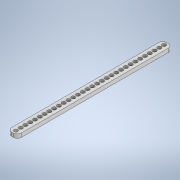
# Autodesk Inventor part: rearLeg_bot
Saved by Autodesk Inventor 2020 (Build 240168000, 168)
## iProperties
Created: 2019-04-04
Part Number: rearLeg_bot
Material: Generic
Document SubType Name: Modeling
Designer: mfans
Density: 1 g/cm^3
Appearance: Default
Author: mfans
Autodesk Inventor part; units mm, degrees
ref_plane "YZ Plane" through (0, 0, 0) normal (1, 0, 0) x (0, 1, 0)
ref_plane "XZ Plane" through (0, 0, 0) normal (0, 1, 0) x (-1, 0, 0)
ref_plane "XY Plane" through (0, 0, 0) normal (0, 0, 1) x (1, 0, 0)
sketch "Sketch1" plane through (0, 0, 0) normal (0, 1, 0) x (-1, 0, 0)
  line L0 (5, 80) -> (-5, 80)
  line L1 (-5, 80) -> (-5, -80)
  line L2 (-5, -80) -> (5, -80)
  line L3 (5, -80) -> (5, 80)
  line L4 (5, 80) -> (-5, -80) construction
  line L5 (-5, 80) -> (5, -80) construction
  point P0 (0, 0)
  dimension "d0" = 10
  dimension "d1" = 160
  constraints: 12 end point, 2 midpoint, 2 parallel, 1 horizontal, 1 perpendicular
  measures "d0" distance of L1.end L2.end
  measures "d1" distance of L0.end L1.end
extrude "Extrusion1" add sketch "Sketch1" along normal blind 4
sketch "Sketch2" plane through (0, 4, 0) normal (0, 1, 0) x (1, 0, 0)
  line L0 (-5, -80) -> (5, -80) projected
  line L1 (-5, 80) -> (-5, -80) projected
  line L2 (-5, -80) -> (5, -80) projected
  line L3 (5, -80) -> (5, 80) projected
  line L4 (5, 80) -> (-5, 80) projected
  point P0 (0, 0)
  point P1 (0, -77.5)
  point P2 (0, -72.5)
  point P3 (0, -67.5)
  point P4 (0, -62.5)
  point P5 (0, -57.5)
  point P6 (0, -52.5)
  point P7 (0, -47.5)
  point P8 (0, -42.5)
  point P9 (0, -37.5)
  point P10 (0, -32.5)
  point P11 (0, -27.5)
  point P12 (0, -22.5)
  point P13 (0, -17.5)
  point P14 (0, -12.5)
  point P15 (0, -7.5)
  point P16 (0, -2.5)
  dimension "d4" = 2.5
  dimension "d7" = 5
  dimension "d24" = 0
  constraints: 1 vertical, 15 other
  measures "d4" distance from line of L0 point (0, -77.5)
  measures "d7" distance of point (0, -77.5) point (0, -72.5)
  measures "d24" horizontal distance of point (0, 0) point (0, -77.5)
hole "Hole1" at (0, 4, 77.5) at (0, 4, 72.5) at (0, 4, 67.5) at (0, 4, 62.5) at (0, 4, 57.5) at (0, 4, 52.5) at (0, 4, 47.5) at (0, 4, 42.5) at (0, 4, 37.5) at (0, 4, 32.5) at (0, 4, 27.5) at (0, 4, 22.5) at (0, 4, 17.5) at (0, 4, 12.5) at (0, 4, 7.5) at (0, 4, 2.5) direction (0, -1, 0) diameter 4 end through all
thicken "Thicken1" operation add thickness 1 both sides no extend neighbours yes toward (0, 0, 1) faces at (-1.6667, 1.3333, 80)
thicken "Thicken2" operation add thickness 1 both sides no extend neighbours yes toward (0, 0, -1) faces at (1.6667, 1.3333, -80)
fillet "Fillet1" radius 4 4 edges at (-5, 2, -81) (5, 2, -81) (5, 2, 81) (-5, 2, 81)
mirror "Mirror1" about plane through (0, 0, 0) normal (0, 0, 1) of "Hole1"
body "Solid1"
